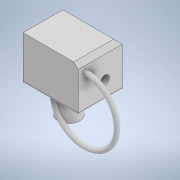
# Autodesk Inventor part: Część1
Saved by Autodesk Inventor 2020 (Build 240168000, 168)
## iProperties
Created: 2020-04-23
Part Number: Część1
Material: Ogólny
Document SubType Name: Modeling
Designer: Marek
Density: 1 g/cm^3
Appearance: Domyślna
Author: Marek
Autodesk Inventor part; units mm, degrees
ref_plane "YZ Plane" through (0, 0, 0) normal (1, 0, 0) x (0, 1, 0)
ref_plane "XZ Plane" through (0, 0, 0) normal (0, 1, 0) x (-1, 0, 0)
ref_plane "XY Plane" through (0, 0, 0) normal (0, 0, 1) x (1, 0, 0)
sketch "Szkic1" plane through (0, 0, 0) normal (0, 1, 0) x (-1, 0, 0)
  circle A0 centre (0, 0) radius 5
  circle A1 centre (0, 0) radius 2
  dimension "d0" = 10
  dimension "d1" = 3
  constraints: 2 centre point, 1 coincident, 1 concentric
  measures "d0" diameter of A0
  measures "d1" radial gap between concentric circles of A0 A1
extrude "Wyciągnięcie proste1" add sketch "Szkic1" along normal blind 10
sketch "Szkic2" plane through (0, 10, 0) normal (0, 1, 0) x (1, 0, 0)
  circle A0 centre (0, 0) radius 5 projected
  circle A1 centre (0, 0) radius 2 projected
  line L0 (-12.5, 11.7523) -> (12.5, 11.7523)
  line L1 (12.5, 11.7523) -> (12.5, -8.2477)
  line L2 (12.5, -8.2477) -> (-12.5, -8.2477)
  line L3 (-12.5, -8.2477) -> (-12.5, 11.7523)
  line L4 (0, 11.1673) -> (0, -8.4509) construction
  dimension "d4" = 20
  dimension "d5" = 25
  constraints: 10 end point, 2 parallel, 1 horizontal, 1 perpendicular, 1 point on line, 1 vertical, 1 other
  measures "d4" distance of L2.end L0.start
  measures "d5" distance of L0.start L0.end
extrude "Wyciągnięcie proste2" add sketch "Szkic2" along normal blind 20 contours A0 | A1 | L0 L1 L2 L3
fillet "Zaokrąglenie1" radius 1 2 edges at (0, 10, 8.2477) (12.5, 10, -1.7523)
chamfer "Faza1" distance 2 angle 45 2 edges at (12.5, 30, -1.7523) (0, 30, -11.7523)
sketch "Szkic3" plane through (12.5, 11, 8.2477) normal (1, 0, 0) x (0, 0, -1)
  line L0 (0, 17) -> (20, 17) projected
  line L1 (0, 0) -> (0, 17) projected
  line L2 (20, 0) -> (0, 0) projected
  line L3 (20, 0) -> (20, 17) projected
  circle A0 centre (2.9885, 14.5933) radius 1.0701
  line L4 (9.4628, 11.1568) -> (9.4628, 6.3913)
  line L5 (7.1085, 8.774) -> (15.0257, 8.774)
  point P0 (8.2477, -11)
  constraints: 4 end point, 1 centre point, 1 horizontal, 1 vertical
revolve "Obrót1" add sketch "Szkic3" angle 360 about axis through (12.5, 11, -11.7523) along (0, 0, 1) contours A0
sketch "Szkic4" plane through (12.5, 11, 8.2477) normal (1, 0, 0) x (0, 0, -1)
  point P0 (8.2477, -11)
  point P1 (12.057, 6.8711)
hole "Otwór1" at (12.5, 17.8711, -3.8093) direction (-1, 0, 0) diameter 3 end through all counterbore diameter 4 counterbore depth 2
